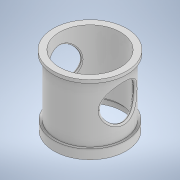
# Autodesk Inventor part: Стакан2
Saved by Autodesk Inventor 2021 (Build 250183000, 183)
## iProperties
Created: 2020-11-15
Part Number: Стакан2
Material: Типовые
Document SubType Name: Modeling
Designer: Тимоха
Density: 1 g/cm^3
Appearance: По умолчанию
Author: Тимоха
Autodesk Inventor part; units mm, degrees
ref_plane "YZ Plane" through (0, 0, 0) normal (1, 0, 0) x (0, 1, 0)
ref_plane "XZ Plane" through (0, 0, 0) normal (0, 1, 0) x (-1, 0, 0)
ref_plane "XY Plane" through (0, 0, 0) normal (0, 0, 1) x (1, 0, 0)
sketch "Эскиз1" plane through (0, 0, 0) normal (0, 0, 1) x (1, 0, 0)
  line L0 (0, 0) -> (70, 0)
  line L1 (70, 0) -> (77.5, 0)
  line L2 (0, 0) -> (0, 150)
  line L3 (77.5, 0) -> (77.5, 20)
  line L4 (77.5, 20) -> (72.5, 20)
  line L5 (72.5, 20) -> (72.5, 143)
  line L6 (65.5, 150) -> (65.5, 15.8104)
  line L7 (65.5, 15.8104) -> (70.5, 10)
  line L8 (70.5, 10) -> (70.5, 0)
  line L9 (72.5, 143) -> (79, 143)
  line L10 (79, 143) -> (79, 150)
  line L11 (79, 150) -> (65.5, 150)
  point P0 (67.5, 0)
  dimension "d0" = 70
  dimension "d1" = 7.5
  dimension "d2" = 150
  dimension "d3" = 20
  dimension "d4" = 5
  dimension "d5" = 123
  dimension "d14" = 6.5
  constraints: 24 end point, 4 perpendicular, 3 vertical, 2 horizontal, 2 point on line, 1 parallel
  measures "d0" distance of L0.start L0.end
  measures "d1" distance of L0.end L1.end
  measures "d2" distance of L0.start L2.end
  measures "d3" distance of L1.end L3.end
  measures "d4" distance of L3.end L4.end
  measures "d5" distance of L4.end L5.end
  measures "d14" distance of L5.end L9.end
revolve "Вращение1" add sketch "Эскиз1" angle 360 about axis through (0, 0, 0) along (0, 1, 0)
sketch "Эскиз2" plane through (0, 0, 0) normal (1, 0, 0) x (0, 1, 0)
  line L0 (0, 0) -> (86.5, 0)
  circle A0 centre (86.5, 0) radius 37
  dimension "d9" = 86.5
  dimension "d10" = 74
  constraints: 2 end point, 1 centre point, 1 coincident, 1 horizontal
  measures "d9" distance of L0.start L0.end
  measures "d10" diameter of A0
extrude "Выдавливание1" cut sketch "Эскиз2" along normal through all both and the other way through all
fillet "Сопряжение1" radius 3 6 edges at (-72.5, 49.5, -0.0038) (-65.5, 49.5001, -0.0781) (54.0486, 86.499, 37) (54.0486, 86.5135, -37) (62.3478, 86.5009, -37) (62.3478, 86.4991, 37)
